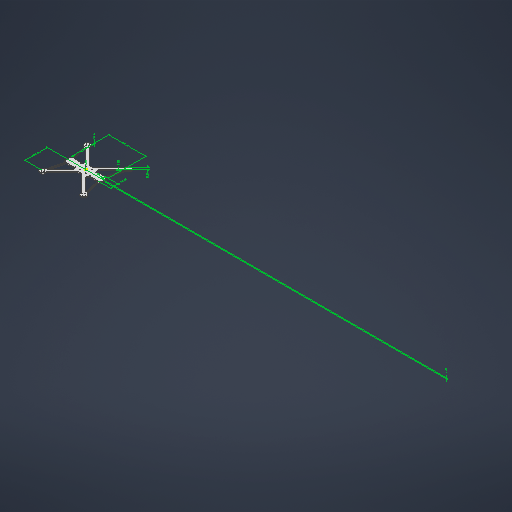
# Autodesk Inventor part: Drone Frame 1.0
Saved by Autodesk Inventor 2026 (Build 300175050, 175E)
## iProperties
Created: 2025-06-14
Part Number: Drone Frame 1.0
Material: Generic
Document SubType Name: Modeling
Designer: User
Density: 1 g/cm^3
Appearance: Default
Author: User
Autodesk Inventor part; units mm, degrees
ref_plane "YZ Plane" through (0, 0, 0) normal (1, 0, 0) x (0, 1, 0)
ref_plane "XZ Plane" through (0, 0, 0) normal (0, 1, 0) x (-1, 0, 0)
ref_plane "XY Plane" through (0, 0, 0) normal (0, 0, 1) x (1, 0, 0)
sketch "Sketch3" plane through (0, 0, 0) normal (0, 1, 0) x (-1, 0, 0)
  line L0 (0, 0) -> (0, -100)
  line L1 (0, 0) -> (125, 0)
  line L2 (0, 0) -> (100, 0)
  line L3 (100, -20) -> (100, 0)
  line L4 (100, 0) -> (32.3997, 0)
  line L5 (100, -20) -> (0, -20)
  line L6 (20, -20) -> (120, -120)
  line L7 (0, -20) -> (100, -120)
  line L8 (120, -120) -> (100, -120)
  dimension "d2" = 100
  dimension "d3" = 125
  dimension "d4" = 20
  dimension "d5" = 100
  dimension "d6" = 100
  dimension "d7" = 45
  dimension "d8" = 20
  dimension "d9" = 100
  constraints: 18 end point, 4 point on line, 2 perpendicular, 1 horizontal, 1 parallel, 1 vertical
  measures "d2" distance of L0.start L0.end
  measures "d3" distance of L0.start L1.end
  measures "d4" distance of L3.start L2.end
  measures "d5" distance of L3.start L5.end
  measures "d6" horizontal distance of L6.start L6.end
  measures "d7" angle of L6 L5
  measures "d8" distance of L5.end L6.start
  measures "d9" horizontal distance of L5.end L7.end
extrude "Body" add sketch "Sketch3" along normal mid plane 5
mirror "Mirror3" about plane through (0, 0, 0) normal (1, 0, 0) of "Body"
mirror "Mirror4" about plane through (0, 0, 0) normal (0, 0, 1) of "Body", "Mirror3"
fillet "Fillet1" radius 5 1 edges at (-100, 0, 20)
fillet "Fillet2" radius 5 1 edges at (-100, 0, -20)
fillet "Fillet3" radius 5 2 edges at (100, 0, 20) (100, 0, -20)
fillet "Fillet4" radius 20 1 edges at (0, 0, 20)
fillet "Fillet5" radius 20 1 edges at (0, 0, -20)
fillet "Fillet6" radius 10 1 edges at (-20, 0, 20)
fillet "Fillet7" radius 10 1 edges at (-20, 0, -20)
fillet "Fillet8" radius 10 1 edges at (20, 0, 20)
fillet "Fillet9" radius 10 1 edges at (20, 0, -20)
sketch "Sketch5" plane through (0, 2.5, 0) normal (0, 1, 0) x (1, 0, 0)
  line L0 (100, 120) -> (120, 120) projected
  circle A0 centre (110, 120) radius 15
  point P0 (0, 0)
  dimension "d31" = 30
  constraints: 1 centre point, 1 midpoint
  measures "d31" diameter of A0
extrude "Circles wins" add sketch "Sketch5" against normal blind 5
mirror "Mirror5" about plane through (0, 0, 0) normal (1, 0, 0) of "Circles wins"
mirror "Mirror6" about plane through (0, 0, 0) normal (0, 0, 1) of "Circles wins", "Mirror5"
sketch "Sketch6" plane through (0, 2.5, 0) normal (0, 1, 0) x (1, 0, 0)
  circle A0 centre (110, 112) radius 1.5
  arc A1 (105.6459, 105.6459) -> (95.6459, 115.6459) centre (110, 120) ccw projected
  circle A2 centre (110, 128) radius 1.5
  circle A3 centre (102, 120) radius 1.5
  circle A4 centre (118, 120) radius 1.5
  circle A5 centre (110, 120) radius 8 construction
  line L0 (102, 120) -> (118, 120) construction
  line L1 (110, 128) -> (110, 112) construction
  line L2 (104.3431, 125.6569) -> (115.6569, 114.3431) construction
  point P0 (0, 0)
  dimension "d54" = 3
  dimension "d55" = 3
  dimension "d56" = 3
  dimension "d57" = 3
  dimension "d59" = 16
  dimension "d149" = 90
  dimension "d150" = 45
  dimension "d151" = 16
  dimension "d153" = 16
  dimension "d154" = 16
  constraints: 6 end point, 6 point on circle, 5 centre point, 1 coincident, 1 perpendicular
  measures "d54" diameter of A2
  measures "d55" diameter of A3
  measures "d56" diameter of A0
  measures "d57" diameter of A4
  measures "d59" distance of L0.start L0.end
  measures "d149" angle of L1 L0
  measures "d150" angle of L1 L2
  measures "d151" distance of L2.start L2.end
  measures "d153" distance of L1.start L1.end
  measures "d154" diameter of A5
extrude "Screw Holes on Circles" cut sketch "Sketch6" against normal blind 5
mirror "Mirror7" about plane through (0, 0, 0) normal (1, 0, 0) of "Screw Holes on Circles"
mirror "Mirror8" about plane through (0, 0, 0) normal (0, 0, 1) of "Screw Holes on Circles", "Mirror7"
sketch "Sketch7" plane through (0, 2.5, 0) normal (0, 1, 0) x (1, 0, 0)
  point P0 (0, 0)
sketch "Sketch8" plane through (0, 2.5, 0) normal (0, 1, 0) x (1, 0, 0)
  line L0 (-95, -20) -> (-44.1421, -20) projected
  line L1 (-89.8962, -20) -> (-110.4466, -105.0066)
  arc A0 (-105.6459, -105.6459) -> (-95.6459, -115.6459) centre (-110, -120) ccw projected
  line L2 (-105.6459, -105.6459) -> (-37.0711, -37.0711) projected
  line L3 (-105.6459, -105.6459) -> (-84.941, -20)
  point P0 (0, 0)
  point P1 (-95.2934, -62.8229)
  point P2 (-92.6536, -20)
  point P3 (-103.4432, -98.4766)
  constraints: 4 end point, 2 point on line, 1 midpoint, 1 parallel, 1 point on circle
extrude "I Beams" add sketch "Sketch8" against normal blind 5
fillet "Fillet10" radius 2 1 edges at (-105.6459, 0, 105.6459)
fillet "Fillet11" radius 5 1 edges at (-84.941, 0, 20)
mirror "Mirror10" about plane through (0, 0, 0) normal (0, 0, 1) of "I Beams", "Fillet10", "Fillet11"
mirror "Mirror11" about plane through (0, 0, 0) normal (1, 0, 0) of "I Beams"
mirror "Mirror12" about plane through (0, 0, 0) normal (0, 0, 1) of "I Beams", "Mirror11"
fillet "Fillet12" radius 5 1 edges at (84.941, 0, 20)
fillet "Fillet13" radius 2 1 edges at (105.6459, 0, 105.6459)
fillet "Fillet14" radius 2 1 edges at (105.6459, 0, -105.6459)
fillet "Fillet15" radius 5 1 edges at (84.941, 0, -20)
sketch "Sketch9" plane through (0, 2.5, 0) normal (0, 1, 0) x (1, 0, 0)
  circle A0 centre (0, 0) radius 22.5 construction
  circle A1 centre (-15.9099, 15.9099) radius 2.5
  circle A2 centre (15.9099, -15.9099) radius 2.5
  line L0 (-15.9099, 15.9099) -> (15.9099, -15.9099) construction
  circle A3 centre (-15.9099, -15.9099) radius 2.5
  circle A4 centre (15.9099, 15.9099) radius 2.5
  line L1 (-15.9099, -15.9099) -> (15.9099, 15.9099) construction
  line L2 (0, 22.5) -> (0, -22.5)
  dimension "d73" = 45
  dimension "d76" = 5
  dimension "d77" = 5
  dimension "d80" = 45
  dimension "d85" = 5
  dimension "d86" = 5
  dimension "d87" = 45
  dimension "d147" = 90
  dimension "d148" = 45
  constraints: 6 end point, 6 point on circle, 5 centre point, 1 coincident, 1 vertical
  measures "d73" diameter of A0
  measures "d76" diameter of A1
  measures "d77" diameter of A2
  measures "d80" distance of L0.start L0.end
  measures "d85" diameter of A3
  measures "d86" diameter of A4
  measures "d87" distance of L1.start L1.end
  measures "d147" angle of L0 L1
  measures "d148" angle of L2 L0
fillet "Fillet16" radius 5 1 edges at (-89.8962, 0, 20)
fillet "Fillet17" radius 5 1 edges at (-89.8962, 0, -20)
fillet "Fillet18" radius 10 1 edges at (-110.4466, 0, -105.0066)
fillet "Fillet19" radius 10 1 edges at (-110.4466, 0, 105.0066)
fillet "Fillet20" radius 5 1 edges at (-95.6459, 0, -115.6459)
fillet "Fillet21" radius 5 1 edges at (95.6459, 0, -115.6459)
fillet "Fillet22" radius 10 1 edges at (110.4466, 0, -105.0066)
fillet "Fillet23" radius 5 1 edges at (89.8962, 0, -20)
fillet "Fillet24" radius 5 1 edges at (89.8962, 0, 20)
fillet "Fillet25" radius 5 1 edges at (110.4466, 0, 105.0066)
fillet "Fillet26" radius 5 1 edges at (95.6459, 0, 115.6459)
fillet "Fillet27" radius 5 1 edges at (-95.6459, 0, 115.6459)
extrude "ESC Holes" cut sketch "Sketch9" against normal blind 5
sketch "Sketch13" plane through (103.9744, -2.5, -98.7321) normal (-0.9719999, 0, -0.2349811) x (-0.2349811, 0, 0.9719999)
  line L0 (3, 1) -> (3, 4)
  line L1 (3, 4) -> (73.0648, 4)
  line L2 (73.0648, 4) -> (73.0648, 1)
  line L3 (73.0648, 1) -> (3, 1)
  line L4 (77.0648, 0) -> (0, 0) projected
  line L5 (0, 5) -> (77.0648, 5) projected
  line L6 (0, 0) -> (0, 5) projected
  line L7 (77.0648, 5) -> (77.0648, 0) projected
  point P0 (120.3996, 2.5)
  point P1 (3, 2.5)
  point P2 (73.0648, 2.5)
  point P3 (-19.0701, 0)
  point P4 (-19.0701, 5)
  dimension "d131" = 3
  dimension "d133" = 1
  dimension "d134" = 1
  dimension "d140" = 4
  constraints: 8 end point, 3 parallel, 2 midpoint, 1 vertical
  measures "d131" distance from line of L6 point (3, 2.5)
  measures "d133" distance between parallel lines of L5 L1
  measures "d134" distance between parallel lines of L4 L3
  measures "d140" distance between parallel lines of L7 L2
extrude "Extrusion7" cut sketch "Sketch13" against normal blind 2 contours L0 L1 L2 L3
chamfer "Chamfer2" distance 2 angle 45 1 edges at (88.7515, 0, -27.2427)
chamfer "Chamfer3" distance 2 angle 45 1 edges at (105.2154, 0, -95.3456)
mirror "Mirror17" about plane through (0, 0, 0) normal (1, 0, 0) of "Extrusion7", "Chamfer2", "Chamfer3"
mirror "Mirror18" about plane through (0, 0, 0) normal (0, 0, 1) of "Extrusion7", "Chamfer2", "Chamfer3", "Mirror17"
sketch "Sketch16" plane through (-91.3706, -2.5, 26.0989) normal (-0.9719999, 0, -0.2349811) x (-0.2349811, 0, 0.9719999)
  line L0 (4.0778, 4) -> (4.0778, 1)
  line L1 (4.0778, 1) -> (59.0778, 1)
  line L2 (59.0778, 1) -> (59.0778, 4)
  line L3 (59.0778, 4) -> (4.0778, 4)
  line L4 (0, 5) -> (74.9083, 5) projected
  line L5 (0, 0) -> (0, 5) projected
  point P0 (-46.8385, 2.5)
  point P1 (37.4541, 5)
  dimension "d167" = 90
  dimension "d168" = 3
  dimension "d169" = 1
  dimension "d170" = 4.0777
  dimension "d171" = 55
  constraints: 8 end point, 2 perpendicular, 1 midpoint, 1 vertical
  measures "d167" angle of L0 L3
  measures "d168" distance of L0.start L0.end
  measures "d169" distance from line of point (37.454, 5) L3
  measures "d170" distance between parallel lines of L5 L0
  measures "d171" distance of L2.end L0.start
extrude "Extrusion9" cut sketch "Sketch16" against normal blind 2
chamfer "Chamfer6" distance 2 angle 45 1 edges at (-90.3829, 0, 30.5329)
chamfer "Chamfer7" distance 2 angle 45 1 edges at (-103.3068, 0, 83.9929)
mirror "Mirror22" about plane through (0, 0, 0) normal (1, 0, 0) of "Extrusion9"
mirror "Mirror23" about plane through (0, 0, 0) normal (0, 0, 1) of "Extrusion9", "Mirror22"
sketch "Sketch17" plane through (0, 2.5, 0) normal (0, 1, 0) x (1, 0, 0)
  circle A0 centre (95, 15) radius 1.75
  line L0 (44.1421, 20) -> (81.0057, 20) projected
  line L1 (100, -15) -> (100, 15) projected
  circle A1 centre (95, -15) radius 1.75
  line L2 (44.1421, -20) -> (81.0057, -20) projected
  circle A2 centre (40, 15) radius 1.75
  circle A3 centre (40, -15) radius 1.75
  line L3 (-100, 15) -> (-100, -15) projected
  line L4 (100, 15) -> (-100, 15) construction
  line L5 (-44.1421, 20) -> (-81.0057, 20) projected
  line L6 (100, -15) -> (-100, -15) construction
  line L7 (40, 15) -> (40, -15) construction
  circle A4 centre (-40, 15) radius 1.75
  circle A5 centre (-40, -15) radius 1.75
  line L8 (-40, 15) -> (-40, -15) construction
  circle A6 centre (-95, 15) radius 1.75
  circle A7 centre (-95, -15) radius 1.75
  point P0 (0, 0)
  point P1 (80.7647, 20)
  point P2 (95, 20)
  point P3 (80.7647, -20)
  point P4 (95, -20)
  point P5 (-80.7647, 20)
  point P6 (-95, 20)
  dimension "d180" = 3.5
  dimension "d181" = 5
  dimension "d182" = 5
  dimension "d183" = 3.5
  dimension "d184" = 5
  dimension "d185" = 5
  dimension "d186" = 3.5
  dimension "d187" = 5
  dimension "d188" = 3.5
  dimension "d190" = 40
  dimension "d191" = 40
  dimension "d192" = 3.5
  dimension "d193" = 3.5
  dimension "d194" = 3.5
  dimension "d195" = 3.5
  dimension "d196" = 30
  dimension "d197" = 5
  constraints: 8 centre point, 8 end point, 6 point on line, 3 perpendicular, 1 horizontal
  measures "d180" diameter of A0
  measures "d181" distance from line of L0 A0.centre
  measures "d182" distance from line of L1 A0.centre
  measures "d183" diameter of A1
  measures "d184" distance from line of L2 A1.centre
  measures "d185" distance from line of A1.centre L1
  measures "d186" diameter of A2
  measures "d187" distance between parallel lines of L4 L5
  measures "d188" diameter of A4
  measures "d190" distance from line of L7 point (0, 0)
  measures "d191" distance from line of point (0, 0) L8
  measures "d192" diameter of A5
  measures "d193" diameter of A3
  measures "d194" diameter of A6
  measures "d195" diameter of A7
  measures "d196" distance of A7.centre A6.centre
  measures "d197" distance from line of A6.centre L3
extrude "Top Holes" cut sketch "Sketch17" against normal blind 5
chamfer "Chamfer8" distance 2 angle 45 1 edges at (90.3829, 0, -30.5329)
chamfer "Chamfer9" distance 2 angle 45 1 edges at (103.3068, 0, -83.9929)
chamfer "Chamfer10" distance 2 angle 45 1 edges at (90.3829, 0, 30.5329)
chamfer "Chamfer11" distance 2 angle 45 1 edges at (103.3068, 0, 83.9929)
body "Solid1"
